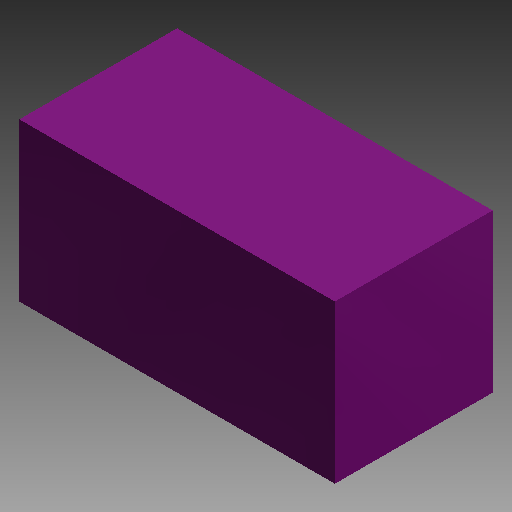
# Autodesk Inventor part: 1nF
Saved by Autodesk Inventor 2018.2 (Build 222227000, 227)
## iProperties
Part Number: 1nF
Material: Generic
Document SubType Name: Modeling
Designer: autocad
Appearance: C0603, 1nF
Author: autocad
Autodesk Inventor part; units mm, degrees
ref_plane "YZ Plane" through (0, 0, 0) normal (1, 0, 0) x (0, 1, 0)
ref_plane "XZ Plane" through (0, 0, 0) normal (0, 1, 0) x (-1, 0, 0)
ref_plane "XY Plane" through (0, 0, 0) normal (0, 0, 1) x (1, 0, 0)
sketch "C0603, 1nF_332" plane through (0, 0, 0) normal (0, 0, 1) x (1, 0, 0)
  line L0 (-0.8, -0.4) -> (-0.8, 0.4)
  line L1 (-0.8, 0.4) -> (0.8, 0.4)
  line L2 (0.8, 0.4) -> (0.8, -0.4)
  line L3 (0.8, -0.4) -> (-0.8, -0.4)
  constraints: 8 end point
extrude "Extrusion1" add sketch "C0603, 1nF_332" along normal blind 0.8
body "Solid1"
